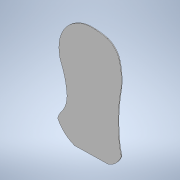
# Autodesk Inventor part: Grundform_Nao_Schuh_original
Saved by Autodesk Inventor 2020.2 (Build 242310000, 310)
## iProperties
Created: 2020-02-10
Part Number: Grundform_Nao_Schuh_original
Material: Generic
Document SubType Name: Modeling
Designer: Mara
Density: 1 g/cm^3
Appearance: Default
Author: Mara
Autodesk Inventor part; units mm, degrees
ref_plane "YZ Plane" through (0, 0, 0) normal (1, 0, 0) x (0, 1, 0)
ref_plane "XZ Plane" through (0, 0, 0) normal (0, 1, 0) x (-1, 0, 0)
ref_plane "XY Plane" through (0, 0, 0) normal (0, 0, 1) x (1, 0, 0)
sketch "Sketch1" plane through (0, 0, 0) normal (0, 0, 1) x (1, 0, 0)
  arc A0 (17, 50.9482) -> (0, 53.5) centre (-5.1444, -38.6736) ccw
  arc A1 (36, 0) -> (33.5994, 33.058) centre (-54.7823, 10.0237) ccw
  line L0 (36, 0) -> (36, -80) construction
  arc A2 (-50, 0) -> (-47.8862, -9) centre (-23.2541, 1.5335) ccw
  line L1 (-50, 0) -> (-51.778, -77.9995) construction
  arc A3 (-39.2282, -46) -> (-47.8862, -9) centre (-148.6597, -52.0939) ccw
  arc A4 (-47.07, -69.156) -> (-39.2282, -46) centre (-76.2937, -46.3536) ccw
  arc A5 (-47.07, -69.156) -> (-51.778, -77.9995) centre (-24.1783, -87.0179) ccw
  line L2 (36, 0) -> (36, -80) construction
  arc A6 (0, 53.5) -> (-50, 0) centre (-4.0952, 7.2128) ccw
  arc A7 (-51.778, -77.9995) -> (-51.8339, -80.4584) centre (-49.0872, -79.2908) ccw
  arc A8 (-51.8339, -80.4584) -> (-28.5899, -101) centre (-14.4772, -61.6088) ccw
  line L3 (-28.5899, -101) -> (18, -100)
  arc A9 (36, 0) -> (33.4774, -67.2753) centre (254.3019, -41.8704) ccw
  arc A10 (18, -100) -> (36, -82.148) centre (8.2499, -72.1685) ccw
  arc A11 (33.4774, -67.2753) -> (36, -80) centre (112.9572, -58.1315) ccw
  arc A12 (36, -82.148) -> (36, -80) centre (32.2206, -81.074) ccw
  arc A13 (33.5994, 33.058) -> (17, 50.9482) centre (8.3724, 26.2971) ccw
  point P0 (0, 0)
  dimension "d6" = 53.5
  dimension "d7" = 50
  dimension "d8" = 36
  dimension "d10" = 80
  dimension "d16" = 77.9995
  dimension "d18" = 9
  dimension "d24" = 4.708
  dimension "d28" = 33.058
  dimension "d29" = 46
  dimension "d34" = 23.1881
  dimension "d35" = 18
  dimension "d36" = 0
  dimension "d38" = 92.317
  dimension "d39" = 91.334
  dimension "d40" = 46.468
  dimension "d41" = 26.7899
  dimension "d42" = 222.281
  dimension "d43" = 80.004
  dimension "d44" = 109.601
  dimension "d45" = 37.0672
  dimension "d46" = 29.0358
  dimension "d48" = 41.843
  dimension "d49" = 29.49
  dimension "d51" = 17
  dimension "d52" = 0
  dimension "d54" = 50
  dimension "d55" = 1.778
  dimension "d56" = 11.8173
  dimension "d57" = 67.2753
  dimension "d58" = 17.852
  dimension "d59" = 20.5416
  dimension "d63" = 26.1172
  dimension "d64" = 101
  dimension "d65" = 100
  dimension "d66" = 3.929
  dimension "d67" = 2.9846
  dimension "d68" = 23.244
  constraints: 28 point on circle, 14 centre point, 9 end point, 4 tangent, 1 collinear, 1 vertical
  measures "d6" distance of point (0, 0) A0.end
  measures "d7" distance of point (0, 0) L1.start
  measures "d8" distance of L0.start point (0, 0)
  measures "d10" distance of L0.start L0.end
  measures "d16" vertical distance of L1.start L1.end
  measures "d18" vertical distance of L1.start A2.end
  measures "d24" horizontal distance of L1.end A4.start
  measures "d28" vertical distance of point (0, 0) A1.end
  measures "d29" vertical distance of A3.start point (0, 0)
  measures "d34" horizontal distance of L1.end L3.start
  measures "d35" horizontal distance of L3.end L0.end
  measures "d36" vertical distance of L0.start point (0, 0)
  measures "d38" radius of A0
  measures "d39" radius of A1
  measures "d40" radius of A6
  measures "d41" radius of A2
  measures "d42" radius of A9
  measures "d43" radius of A11
  measures "d44" radius of A3
  measures "d45" radius of A4
  measures "d46" radius of A5
  measures "d48" radius of A8
  measures "d49" radius of A10
  measures "d51" horizontal distance of A0.end A0.start
  measures "d52" horizontal distance of point (0, 0) A0.end
  measures "d54" distance of point (0, 0) L1.start
  measures "d55" horizontal distance of L1.start L1.end
  measures "d56" distance from line of L1 A3.start
  measures "d57" vertical distance of L0.start A9.end
  measures "d58" vertical distance of L3.end A10.end
  measures "d59" vertical distance of A7.end L3.start
  measures "d63" radius of A13
  measures "d64" vertical distance of L3.start point (0, 0)
  measures "d65" vertical distance of L3.end point (0, 0)
  measures "d66" radius of A12
  measures "d67" radius of A7
  measures "d68" horizontal distance of L3.start A7.end
extrude "Extrusion1" add sketch "Sketch1" along normal blind 1
body "Solid1"
